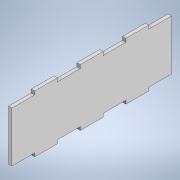
# Autodesk Inventor part: voorkant
Saved by Autodesk Inventor 2022 (Build 260153000, 153)
## iProperties
Created: 2022-01-28
Part Number: voorkant
Material: Generic
Document SubType Name: Modeling
Designer: keemi
Density: 1 g/cm^3
Appearance: Default
Author: keemi
Autodesk Inventor part; units mm, degrees
ref_plane "YZ Plane" through (0, 0, 0) normal (1, 0, 0) x (0, 1, 0)
ref_plane "XZ Plane" through (0, 0, 0) normal (0, 1, 0) x (-1, 0, 0)
ref_plane "XY Plane" through (0, 0, 0) normal (0, 0, 1) x (1, 0, 0)
sketch "Sketch1" plane through (0, 0, 0) normal (1, 0, 0) x (0, 1, 0)
  line L0 (0, 0) -> (0, -140)
  line L1 (0, -140) -> (3, -140)
  line L2 (3, -140) -> (3, -120)
  line L3 (3, -120) -> (3, -100)
  line L4 (3, -100) -> (3, -80)
  line L5 (3, -80) -> (3, -60)
  line L6 (3, -60) -> (3, -40)
  line L7 (3, -40) -> (3, -20)
  line L8 (3, -20) -> (3, 0)
  line L9 (0, 0) -> (3, 0)
  line L10 (3, -20) -> (-0.6185, -20)
  line L11 (3, -40) -> (0, -40)
  line L12 (3, -60) -> (0, -60)
  line L13 (3, -80) -> (0, -80)
  line L14 (3, -100) -> (0, -100)
  line L15 (3, -120) -> (0, -120)
  line L16 (0, 0) -> (25, 0)
  line L17 (25, 0) -> (0, 0)
  line L18 (0, 0) -> (0, -140)
  line L19 (0, -140) -> (25, -140)
  line L20 (25, -140) -> (25, 0)
  point P0 (0, -20)
  dimension "d1" = 140
  dimension "d2" = 3
  dimension "d3" = 20
  dimension "d4" = 20
  dimension "d5" = 20
  dimension "d6" = 20
  dimension "d7" = 20
  dimension "d8" = 20
  dimension "d9" = 20
  dimension "d10" = 25
  constraints: 42 end point, 12 point on line, 7 perpendicular, 3 horizontal, 2 parallel, 1 vertical
  measures "d1" distance of L0.start L0.end
  measures "d2" distance of L0.end L1.end
  measures "d3" distance of L1.end L2.end
  measures "d4" distance of L2.end L3.end
  measures "d5" distance of L3.end L4.end
  measures "d6" distance of L4.end L5.end
  measures "d7" distance of L5.end L6.end
  measures "d8" distance of L6.end L7.end
  measures "d9" distance of L7.end L8.end
  measures "d10" distance of L0.start L16.end
extrude "Extrusion1" add sketch "Sketch1" along normal blind 3 contours L0 L10 L7 L11 | L12 L5 L13 L0 | L7 L8 L16 L20 L19 L2 L3 L4 L5 L6 | L14 L3 L15 L0
mirror "Mirror1" about plane through (0, 25, -140) normal (0, 1, 0) of "Extrusion1"
body "Solid1"
